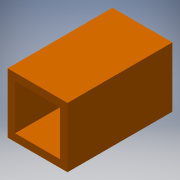
# Autodesk Inventor part: 2018 Cube Back Stop Vertical
Saved by Autodesk Inventor 2018 (Build 220112000, 112)
## iProperties
Created: 2018-01-23
Part Number: 2018 Cube Back Stop Vertical
Material: Generic
Document SubType Name: Modeling
Designer: Apple
Density: 1 g/cm^3
Appearance: Default
Author: Apple
Autodesk Inventor part; units mm, degrees
ref_plane "YZ Plane" through (0, 0, 0) normal (1, 0, 0) x (0, 1, 0)
ref_plane "XZ Plane" through (0, 0, 0) normal (0, 1, 0) x (-1, 0, 0)
ref_plane "XY Plane" through (0, 0, 0) normal (0, 0, 1) x (1, 0, 0)
sketch "Sketch1" plane through (0, 0, 0) normal (0, 0, 1) x (1, 0, 0)
  line L0 (-22.225, -63.5) -> (-3.175, -63.5) projected
  line L1 (0, -63.5) -> (-25.4, -63.5)
  line L2 (-25.4, -63.5) -> (-25.4, -88.9)
  line L3 (-25.4, -88.9) -> (0, -88.9)
  line L4 (0, -88.9) -> (0, -63.5)
  line L5 (-22.225, -85.725) -> (-22.225, -66.675)
  line L6 (-22.225, -66.675) -> (-3.175, -66.675)
  line L7 (-3.175, -66.675) -> (-3.175, -85.725)
  line L8 (-3.175, -85.725) -> (-22.225, -85.725)
  point P0 (0, 0)
  dimension "d0" = 25.4
  dimension "d1" = 25.4
  dimension "d2" = 3.175
  constraints: 16 end point, 4 parallel, 2 perpendicular, 1 horizontal, 1 point on line, 3 other
  measures "d0" distance of L3.end L1.start
  measures "d1" distance of L2.end L3.end
  measures "d2" distance between parallel lines of L2 L5
extrude "Extrusion1" add sketch "Sketch1" along normal blind 44.45
body "Solid1"
